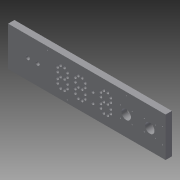
# Autodesk Inventor part: licht_200_top1_teil_b
Saved by Autodesk Inventor 2015 (Build 190159000, 159)
## iProperties
Created: 2018-01-11
Part Number: licht_200_top1_teil_b
Material: Generisch
Document SubType Name: Blech
Designer: schueler
Density: 1 g/cm^3
Sheet Metal Rule: Standard_mm
Appearance: Vorgabe
Author: schueler
Autodesk Inventor part; units mm, degrees
ref_plane "YZ Plane" through (0, 0, 0) normal (1, 0, 0) x (0, 1, 0)
ref_plane "XZ Plane" through (0, 0, 0) normal (0, 1, 0) x (-1, 0, 0)
ref_plane "XY Plane" through (0, 0, 0) normal (0, 0, 1) x (1, 0, 0)
sketch "Skizze1" plane through (0, 0, 0) normal (0, 1, 0) x (-1, 0, 0)
  line L0 (0, 0) -> (400, 0)
  line L1 (400, -100) -> (0, -100)
  line L2 (0, -100) -> (0, 0)
  line L3 (100, 0) -> (100, -100) construction
  line L4 (0, -92) -> (400, -92) construction
  circle A0 centre (100, -8) radius 1.5
  line L5 (8, 0) -> (8, -100) construction
  circle A1 centre (8, -30) radius 1.5
  circle A2 centre (8, -70) radius 1.5
  line L6 (400, -8) -> (0, -8) construction
  circle A3 centre (250, -92) radius 1.5
  line L7 (300, 0) -> (300, -100) construction
  circle A4 centre (300, -8) radius 1.5
  line L8 (400, -100) -> (400, 0)
  line L9 (250, -8) -> (250, -92) construction
  point P0 (100, -92)
  point P1 (100, -8)
  point P2 (300, -92)
  dimension "d2" = 400
  dimension "d7" = 100
  dimension "d16" = 3
  dimension "d19" = 8
  dimension "d23" = 3
  dimension "d24" = 3
  dimension "d46" = 30
  dimension "d47" = 30
  dimension "d57" = 8
  dimension "d58" = 3
  dimension "d63" = 200
  dimension "d69" = 3
  dimension "d116" = 250
  dimension "d127" = 100
  dimension "d128" = 8
  constraints: 22 point on line, 21 end point, 5 centre point, 5 perpendicular, 1 coincident, 1 horizontal, 1 parallel, 1 vertical
  measures "d2" distance of L1.start L1.end
  measures "d7" distance of L0.start L3.start
  measures "d16" diameter of A0
  measures "d19" distance of L0.start L5.start
  measures "d23" diameter of A1
  measures "d24" diameter of A2
  measures "d46" distance from line of L0 A1.centre
  measures "d47" distance from line of L1 A2.centre
  measures "d57" distance between parallel lines of L0 L6
  measures "d58" diameter of A3
  measures "d63" distance between parallel lines of L3 L7
  measures "d69" diameter of A4
  measures "d116" distance from line of L2 L9.start
  measures "d127" distance between parallel lines of L0 L1
  measures "d128" distance between parallel lines of L1 L4
extrude "Extrusion9" add sketch "Skizze1" along normal blind 16
sketch "Skizze6" plane through (0, 0, 0) normal (0, -1, 0) x (1, 0, 0)
  line L0 (-400, -100) -> (0, -100) construction
  line L1 (0, -100) -> (0, 0) construction
  line L2 (0, 0) -> (-400, 0) construction
  line L3 (-400, 0) -> (-400, -100) construction
  line L4 (0, -50) -> (-400, -50) construction
  line L5 (-400, 0) -> (-400, -100) construction
  line L6 (0, 0) -> (-400, 0) construction
  line L7 (-400, -100) -> (0, -100) construction
  line L8 (-250, 0) -> (-250, -100) construction
  line L9 (-257.5, 0) -> (-257.5, -100) construction
  line L10 (-267.5, 0) -> (-267.5, -100) construction
  line L11 (-275, 0) -> (-275, -100) construction
  line L12 (-230, 0) -> (-230, -100) construction
  line L13 (-222.5, 0) -> (-222.5, -100) construction
  line L14 (-212.5, 0) -> (-212.5, -100) construction
  line L15 (-205, 0) -> (-205, -102.7121) construction
  line L16 (-165, 0) -> (-165, -100) construction
  line L17 (-157.5, 0) -> (-157.5, -100) construction
  line L18 (-147.5, 0) -> (-147.5, -100) construction
  line L19 (-140, 0) -> (-140, -100) construction
  line L20 (-275, -42.5) -> (-140, -42.5) construction
  line L21 (-140, -32.5) -> (-275, -32.5) construction
  line L22 (-275, -25) -> (-140, -25) construction
  line L23 (-275, -57.5) -> (-140, -57.5) construction
  line L24 (-140, -67.5) -> (-275, -67.5) construction
  line L25 (-275, -75) -> (-140, -75) construction
  line L26 (-240, 0) -> (-240, -100) construction
  line L27 (-185, -67.5) -> (-185, -42.5) construction
  point P0 (-267.5, -75)
  point P1 (-257.5, -75)
  point P2 (-250, -67.5)
  point P3 (-250, -57.5)
  point P4 (-257.5, -50)
  point P5 (-267.5, -50)
  point P6 (-267.5, -25)
  point P7 (-257.5, -25)
  point P8 (-250, -32.5)
  point P9 (-250, -42.5)
  point P10 (-230, -42.5)
  point P11 (-230, -32.5)
  point P12 (-222.5, -25)
  point P13 (-212.5, -25)
  point P14 (-205, -32.5)
  point P15 (-205, -42.5)
  point P16 (-222.5, -50)
  point P17 (-230, -57.5)
  point P18 (-230, -67.5)
  point P19 (-222.5, -75)
  point P20 (-212.5, -75)
  point P21 (-205, -67.5)
  point P22 (-205, -57.5)
  point P23 (-212.5, -50)
  point P24 (-157.5, -25)
  point P25 (-147.5, -25)
  point P26 (-165, -32.5)
  point P27 (-165, -42.5)
  point P28 (-157.5, -50)
  point P29 (-147.5, -50)
  point P30 (-147.5, -75)
  point P31 (-157.5, -75)
  point P32 (-165, -67.5)
  point P33 (-165, -57.5)
  point P34 (-350, -50)
  point P35 (-325, -50)
  dimension "d137" = 7.5
  dimension "d138" = 10
  dimension "d139" = 7.5
  dimension "d141" = 7.5
  dimension "d142" = 10
  dimension "d143" = 7.5
  dimension "d144" = 40
  dimension "d145" = 7.5
  dimension "d146" = 10
  dimension "d147" = 7.5
  dimension "d148" = 7.5
  dimension "d149" = 10
  dimension "d150" = 7.5
  dimension "d151" = 7.5
  dimension "d152" = 10
  dimension "d153" = 7.5
  dimension "d156" = 50
  dimension "d157" = 25
  dimension "d180" = 240
  dimension "d181" = 10
  dimension "d182" = 10
  dimension "d201" = 20
  constraints: 72 point on line, 50 end point, 12 perpendicular, 8 coincident, 8 midpoint, 8 parallel, 3 vertical, 1 horizontal, 27 other
  measures "d137" distance between parallel lines of L12 L13
  measures "d138" distance between parallel lines of L14 L13
  measures "d139" distance between parallel lines of L15 L14
  measures "d141" distance between parallel lines of L9 L8
  measures "d142" distance between parallel lines of L10 L9
  measures "d143" distance between parallel lines of L10 L11
  measures "d144" distance between parallel lines of L16 L15
  measures "d145" distance between parallel lines of L17 L16
  measures "d146" distance between parallel lines of L18 L17
  measures "d147" distance between parallel lines of L19 L18
  measures "d148" distance between parallel lines of L4 L20
  measures "d149" distance between parallel lines of L20 L21
  measures "d150" distance between parallel lines of L21 L22
  measures "d151" distance between parallel lines of L4 L23
  measures "d152" distance between parallel lines of L23 L24
  measures "d153" distance between parallel lines of L24 L25
  measures "d156" distance from line of L3 point (-350, -50)
  measures "d157" distance of point (-350, -50) point (-325, -50)
  measures "d180" distance between parallel lines of L1 L26
  measures "d181" distance between parallel lines of L26 L8
  measures "d182" distance between parallel lines of L12 L26
  measures "d201" distance between parallel lines of L15 L27
hole "Bohrung5" at (-267.5, 0, -75) at (-257.5, 0, -75) at (-250, 0, -67.5) at (-250, 0, -57.5) at (-257.5, 0, -50) at (-267.5, 0, -50) at (-275, 0, -57.5) at (-275, 0, -67.5) at (-275, 0, -42.5) at (-275, 0, -32.5) at (-267.5, 0, -25) at (-257.5, 0, -25) at (-250, 0, -32.5) at (-250, 0, -42.5) at (-230, 0, -42.5) at (-230, 0, -32.5) at (-222.5, 0, -25) at (-212.5, 0, -25) at (-205, 0, -32.5) at (-205, 0, -42.5) at (-222.5, 0, -50) at (-230, 0, -57.5) at (-230, 0, -67.5) at (-222.5, 0, -75) at (-212.5, 0, -75) at (-205, 0, -67.5) at (-205, 0, -57.5) at (-212.5, 0, -50) at (-157.5, 0, -25) at (-147.5, 0, -25) at (-165, 0, -32.5) at (-165, 0, -42.5) at (-157.5, 0, -50) at (-147.5, 0, -50) at (-140, 0, -57.5) at (-140, 0, -67.5) at (-147.5, 0, -75) at (-157.5, 0, -75) at (-165, 0, -67.5) at (-165, 0, -57.5) at (-140, 0, -42.5) at (-140, 0, -32.5) at (-185, 0, -42.5) at (-185, 0, -67.5) direction (0, 1, 0) diameter 6 depth 30 tip angle 118 counterbore diameter 8 counterbore depth 12
hole "Bohrung6" at (-350, 0, -50) at (-325, 0, -50) direction (0, 1, 0) diameter 7 depth 30 tip angle 118 counterbore diameter 10 counterbore depth 12
sketch "Skizze7" plane through (0, 16, 0) normal (0, 1, 0) x (1, 0, 0)
  circle A0 centre (-250, 92) radius 1.5 projected
  circle A1 centre (-300, 8) radius 1.5 projected
  circle A2 centre (-8, 70) radius 1.5 projected
  circle A3 centre (-8, 30) radius 1.5 projected
  circle A4 centre (-100, 8) radius 1.5 projected
  line L0 (0, 0) -> (-400, 0) construction
  line L1 (-400, 0) -> (-400, 100) construction
  line L2 (-400, 100) -> (0, 100) construction
  line L3 (0, 100) -> (0, 0) construction
  line L4 (-40, 50) -> (0, 50) construction
  line L5 (0, 0) -> (0, 100) construction
  line L6 (-25.4, 35.4) -> (-54.6, 35.4) construction
  line L7 (-54.6, 35.4) -> (-54.6, 64.6) construction
  line L8 (-54.6, 64.6) -> (-25.4, 64.6) construction
  line L9 (-25.4, 64.6) -> (-25.4, 35.4) construction
  line L10 (-40, 50) -> (-40, 100) construction
  circle A5 centre (-40, 50) radius 25.4 construction
  line L11 (-100, 0) -> (-100, 100) construction
  line L12 (-85.4, 35.4) -> (-114.6, 35.4) construction
  line L13 (-114.6, 35.4) -> (-114.6, 64.6) construction
  line L14 (-114.6, 64.6) -> (-85.4, 64.6) construction
  line L15 (-85.4, 64.6) -> (-85.4, 35.4) construction
  circle A6 centre (-100, 50) radius 25.4 construction
  point P0 (-54.6, 50)
  point P1 (-40, 64.6)
  point P2 (-100, 35.4)
  dimension "d184" = 40
  dimension "d185" = 29.2
  dimension "d186" = 29.2
  dimension "d202" = 50.8
  dimension "d203" = 60
  dimension "d204" = 29.2
  dimension "d205" = 29.2
  dimension "d206" = 50.8
  constraints: 30 end point, 10 coincident, 6 parallel, 6 perpendicular, 6 point on line, 5 midpoint, 3 horizontal, 2 centre point, 1 collinear
  measures "d184" distance between parallel lines of L3 L10
  measures "d185" distance of L6.start L6.end
  measures "d186" distance between parallel lines of L8 L6
  measures "d202" diameter of A5
  measures "d203" distance between parallel lines of L11 L10
  measures "d204" distance of L12.start L12.end
  measures "d205" distance of L12.end L13.end
  measures "d206" diameter of A6
hole "Bohrung7" at (-100, 16, -8) at (-250, 16, -92) at (-300, 16, -8) at (-8, 16, -70) at (-8, 16, -30) direction (0, -1, 0) diameter 3 depth 8 tip angle 118 countersink diameter 8 countersink angle 90
hole "Bohrung8" at (-40, 16, -50) at (-100, 16, -50) direction (0, -1, 0) diameter 24 end through all
hole "Bohrung9" at (-54.6, 16, -64.6) at (-25.4, 16, -35.4) at (-25.4, 16, -64.6) at (-54.6, 16, -35.4) at (-85.4, 16, -35.4) at (-85.4, 16, -64.6) at (-114.6, 16, -64.6) at (-114.6, 16, -35.4) direction (0, -1, 0) diameter 3 end through all
sketch "Skizze9" plane through (0, 16, 0) normal (0, 1, 0) x (1, 0, 0)
  circle A0 centre (-100, 50) radius 12 projected
  line L0 (-82.5, 42.5) -> (-117.5, 42.5)
  line L1 (-117.5, 42.5) -> (-117.5, 57.5)
  line L2 (-117.5, 57.5) -> (-82.5, 57.5)
  line L3 (-82.5, 57.5) -> (-82.5, 42.5)
  line L4 (-100, 50) -> (-100, 42.5) construction
  line L5 (-100, 50) -> (-117.5, 50) construction
  point P0 (0, 0)
  dimension "d211" = 15
  dimension "d212" = 35
  constraints: 12 end point, 2 midpoint, 2 parallel, 2 perpendicular, 1 horizontal, 1 vertical
  measures "d211" distance of L0.end L1.end
  measures "d212" distance of L0.start L0.end
extrude "Extrusion11" cut sketch "Skizze9" against normal blind 2 contours A0 L0 L2 | A0 L2 L3 L0 | A0 L0 L1 L2
equation "\"Biegeradius\" = Stärke"
equation "\"BreiteBiegungsfreistellung\" = Stärke"
equation "\"TiefeBiegungsfreistellung\" = 0.5 * Stärke"
equation "\"GrößeEckenfreistellung\" = 4 * Stärke"
equation "\"MinimalRest\" = 2 * Stärke"
equation "\"Übergangsradius\" = Biegeradius"
equation "\"JacobiRadiusGröße\" = Biegeradius"
equation "\"Abstandsgröße\" = Stärke"
equation "\"Stärke\" = 0.5"
